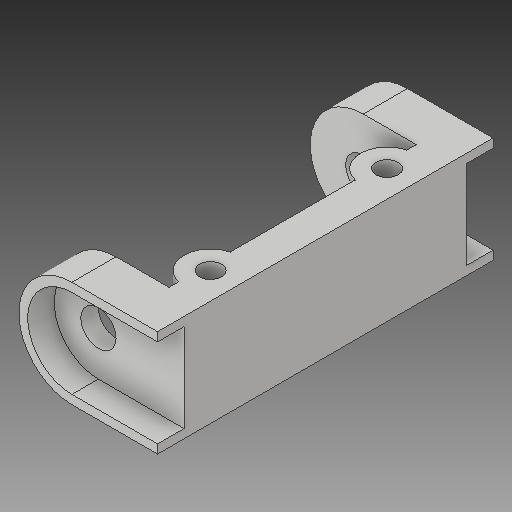
# Autodesk Inventor part: Steering_Arm
Saved by Autodesk Inventor 2019 (Build 230136000, 136)
## iProperties
Created: 2019-03-03
Part Number: Steering_Arm
Material: Generic
Document SubType Name: Modeling
Designer: alarr
Density: 1 g/cm^3
Appearance: Default
Author: alarr
Autodesk Inventor part; units mm, degrees
ref_plane "YZ Plane" through (0, 0, 0) normal (1, 0, 0) x (0, 1, 0)
ref_plane "XZ Plane" through (0, 0, 0) normal (0, 1, 0) x (-1, 0, 0)
ref_plane "XY Plane" through (0, 0, 0) normal (0, 0, 1) x (1, 0, 0)
sketch "Sketch1" plane through (0, 0, 0) normal (0, 0, 1) x (1, 0, 0)
  line L0 (-79.121, 7.62) -> (-79.121, -7.62) projected
  line L1 (-79.121, -7.62) -> (-84.201, -7.62) projected
  line L2 (-84.201, 7.62) -> (-79.121, 7.62) projected
  line L3 (-80.391, -7.62) -> (-92.71, -7.62)
  line L4 (-92.71, -7.62) -> (-92.71, 7.62) construction
  line L5 (-92.71, 7.62) -> (-80.391, 7.62)
  line L6 (-80.391, 7.62) -> (-80.391, -7.62)
  arc A0 (-92.71, 7.62) -> (-92.71, -7.62) centre (-92.71, 0) ccw
  arc A1 (-92.71, -7.62) -> (-92.71, 7.62) centre (-92.71, 0) ccw construction
  line L7 (-92.71, 0) -> (-100.33, 0) construction
  point P0 (0, 0)
  dimension "d0" = 1.27
  dimension "d1" = 19.939
  constraints: 10 end point, 5 point on circle, 2 centre point, 2 parallel, 2 point on line, 1 horizontal, 1 midpoint, 1 perpendicular
  measures "d0" distance between parallel lines of L0 L6
  measures "d1" distance from line of L6 L7.end
extrude "Extrusion1" add sketch "Sketch1" along normal mid plane 48.26 contours L6 L1 L3 A0 L5 L2
sketch "Sketch2" plane through (-92.71, 7.62, 24.13) normal (0, 1, 0) x (1, 0, 0)
  circle A0 centre (8.509, 11.43) radius 1.5875 projected
  circle A1 centre (8.509, 36.83) radius 1.5875 projected
  circle A2 centre (8.509, 11.43) radius 1.5875
  circle A3 centre (8.509, 36.83) radius 1.5875
  point P0 (92.71, 24.13)
  constraints: 2 centre point, 2 coincident, 2 concentric
extrude "Extrusion2" cut sketch "Sketch2" against normal through all
sketch "Sketch3" plane through (-92.71, 7.62, 24.13) normal (0, 1, 0) x (1, 0, 0)
  line L0 (0, 48.26) -> (-7.62, 48.26) projected
  line L1 (0, 48.26) -> (12.319, 48.26) projected
  line L2 (-7.62, 0) -> (0, 0) projected
  line L3 (12.319, 0) -> (0, 0) projected
  circle A0 centre (8.509, 11.43) radius 1.5875 projected
  circle A1 centre (8.509, 36.83) radius 1.5875 projected
  line L4 (12.319, 48.26) -> (12.319, 0) projected
  arc A2 (7.62, 15.1348) -> (7.62, 7.7252) centre (8.509, 11.43) ccw
  circle A3 centre (8.509, 36.83) radius 1.5875 projected
  arc A4 (7.62, 40.5348) -> (7.62, 33.1252) centre (8.509, 36.83) ccw
  line L5 (-7.62, 48.26) -> (-7.62, 0) projected
  line L6 (-7.62, 24.13) -> (12.319, 24.13) construction
  line L7 (-7.62, 41.91) -> (7.62, 41.91)
  line L8 (7.62, 41.91) -> (7.62, 40.5348)
  line L9 (7.62, 6.35) -> (-7.62, 6.35)
  line L10 (-7.62, 6.35) -> (-7.62, 41.91)
  line L11 (-7.62, 41.91) -> (7.62, 6.35) construction
  line L12 (7.62, 41.91) -> (-7.62, 6.35) construction
  line L13 (7.62, 40.5348) -> (7.62, 33.1252) construction
  arc A5 (12.319, 36.83) -> (7.62, 40.5348) centre (8.509, 36.83) ccw construction
  arc A6 (7.62, 33.1252) -> (12.319, 36.83) centre (8.509, 36.83) ccw construction
  line L14 (7.62, 33.1252) -> (7.62, 15.1348)
  line L15 (7.62, 15.1348) -> (7.62, 7.7252) construction
  arc A7 (12.319, 11.43) -> (7.62, 15.1348) centre (8.509, 11.43) ccw construction
  arc A8 (7.62, 7.7252) -> (12.319, 11.43) centre (8.509, 11.43) ccw construction
  line L16 (7.62, 7.7252) -> (7.62, 6.35)
  point P0 (92.71, 24.13)
  point P1 (0, 24.13)
  dimension "d17" = 35.56
  dimension "d18" = 15.24
  constraints: 22 end point, 12 point on circle, 6 centre point, 6 parallel, 5 perpendicular, 4 midpoint, 4 point on line, 4 tangent, 2 coincident, 1 horizontal
  measures "d17" distance between parallel lines of L7 L9
  measures "d18" distance of L7.start L7.end
extrude "Extrusion3" cut sketch "Sketch3" against normal through all contours L7 L8 A4 L14 A2 L16 L9 L5
sketch "Sketch4" plane through (0, 0, 0) normal (0, 0, 1) x (1, 0, 0)
  arc A0 (-92.71, 7.62) -> (-92.71, -7.62) centre (-92.71, 0) ccw projected
  circle A1 centre (-92.71, 0) radius 2.54
  point P0 (0, 0)
  dimension "d11" = 5.08
  constraints: 1 centre point, 1 coincident
  measures "d11" diameter of A1
extrude "Extrusion4" cut sketch "Sketch4" along normal mid plane 43.18
sketch "Sketch5" plane through (0, 0, 24.13) normal (0, 0, 1) x (1, 0, 0)
  line L0 (-80.391, -7.62) -> (-80.391, 7.62) projected
  line L1 (-80.391, 7.62) -> (-92.71, 7.62) projected
  arc A0 (-92.71, 7.62) -> (-92.71, -7.62) centre (-92.71, 0) ccw projected
  line L2 (-92.71, -7.62) -> (-80.391, -7.62) projected
  arc A1 (-92.71, 6.35) -> (-92.71, -6.35) centre (-92.71, 0) ccw
  line L3 (-92.71, 6.35) -> (-81.661, 6.35)
  line L4 (-81.661, 6.35) -> (-81.661, -6.35) construction
  line L5 (-81.661, -6.35) -> (-92.71, -6.35)
  line L6 (-81.661, 6.35) -> (-80.391, 6.35)
  line L7 (-81.661, -6.35) -> (-80.391, -6.35)
  line L8 (-80.391, 7.62) -> (-80.391, -7.62) projected
  point P0 (0, 0)
  dimension "d14" = 1.27
  constraints: 10 end point, 2 point on circle, 2 point on line, 1 centre point, 1 parallel, 1 perpendicular, 3 other
  measures "d14" radial gap between concentric circles of A0 A1
extrude "Extrusion5" cut sketch "Sketch5" against normal blind 3.81 contours L7 L5 A1 L3 L6 L0
mirror "Mirror1" about plane through (0, 0, 0) normal (0, 0, 1) of "Extrusion5"
body "Solid1"
